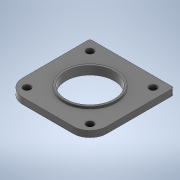
# Autodesk Inventor part: soportemotor
Saved by Autodesk Inventor 2020.2 (Build 242310000, 310)
## iProperties
Created: 2021-01-03
Part Number: soportemotor
Material: Generic
Document SubType Name: Modeling
Designer: JK
Density: 1 g/cm^3
Appearance: Smooth - Black
Author: JK
Autodesk Inventor part; units mm, degrees
ref_plane "YZ Plane" through (0, 0, 0) normal (1, 0, 0) x (0, 1, 0)
ref_plane "XZ Plane" through (0, 0, 0) normal (0, 1, 0) x (-1, 0, 0)
ref_plane "XY Plane" through (0, 0, 0) normal (0, 0, 1) x (1, 0, 0)
sketch "Sketch1" plane through (0, 0, 0) normal (0, 1, 0) x (-1, 0, 0)
  line L0 (-20, 20) -> (20, 20)
  line L1 (20, 20) -> (20, -20)
  line L2 (20, -20) -> (-20, -20)
  line L3 (-20, -20) -> (-20, 20)
  line L4 (-20, 20) -> (20, -20) construction
  line L5 (20, 20) -> (-20, -20) construction
  circle A0 centre (0, 0) radius 4
  circle A1 centre (0, 8.5) radius 1.75
  circle A2 centre (0, -8.5) radius 1.75
  point P0 (0, 0)
  point P1 (0, 0)
  dimension "d0" = 40
  dimension "d1" = 40
  dimension "d2" = 8
  dimension "d3" = 3.5
  dimension "d4" = 3.5
  dimension "d5" = 8.5
  dimension "d6" = 8.5
  constraints: 12 end point, 4 midpoint, 3 centre point, 2 coincident, 2 parallel, 2 vertical alignment, 1 horizontal, 1 perpendicular
  measures "d0" distance of L0.end L1.end
  measures "d1" distance of L1.end L2.end
  measures "d2" diameter of A0
  measures "d3" diameter of A1
  measures "d4" diameter of A2
  measures "d5" distance of point (0, 0) A2.centre
  measures "d6" distance of point (0, 0) A1.centre
extrude "Extrusion1" add sketch "Sketch1" along normal blind 3
chamfer "Chamfer1" distance 2 angle 45 2 edges at (1.75, 3, -8.5) (1.75, 3, 8.5)
sketch "Sketch3" plane through (0, 3, 0) normal (0, 1, 0) x (1, 0, 0)
  circle A0 centre (-15, -15) radius 1.75
  circle A1 centre (-15, 15) radius 1.75
  circle A2 centre (15, 15) radius 1.75
  circle A3 centre (15, -15) radius 1.75
  point P0 (0, 0)
  dimension "d13" = 3.5
  dimension "d14" = 15
  dimension "d15" = 15
  dimension "d16" = 15
  dimension "d17" = 15
  constraints: 4 centre point, 3 equal radius, 2 horizontal alignment, 2 vertical alignment
  measures "d13" diameter of A0
  measures "d14" horizontal distance of A0.centre point (0, 0)
  measures "d15" horizontal distance of A0.centre point (0, 0)
  measures "d16" horizontal distance of point (0, 0) A3.centre
  measures "d17" horizontal distance of point (0, 0) A1.centre
extrude "Extrusion2" cut sketch "Sketch3" against normal through all
sketch "Sketch4" plane through (0, 3, 0) normal (0, 1, 0) x (1, 0, 0)
  circle A0 centre (0, 0) radius 11.5
  dimension "d20" = 23
  constraints: 1 centre point, 1 coincident
  measures "d20" diameter of A0
extrude "Extrusion3" cut sketch "Sketch4" against normal blind 10
sketch "Sketch5" plane through (0, 3, 0) normal (0, 1, 0) x (1, 0, 0)
  circle A0 centre (0, 0) radius 11.5
  circle A1 centre (0, 0) radius 12.5
  arc A2 (2.6001, -11.2022) -> (2.6001, 11.2022) centre (0, 0) ccw projected
  dimension "d23" = 1
  constraints: 2 centre point, 2 coincident, 1 concentric
  measures "d23" radial gap between concentric circles of A1 A0
extrude "Extrusion4" add sketch "Sketch5" along normal mid plane 2
fillet "Fillet2" radius 8 2 edges at (-20, 1.5, 20) (20, 1.5, 20)
fillet "Fillet3" radius 1 2 edges at (20, 1.5, -20) (-20, 1.5, -20)
body "Solid1"
